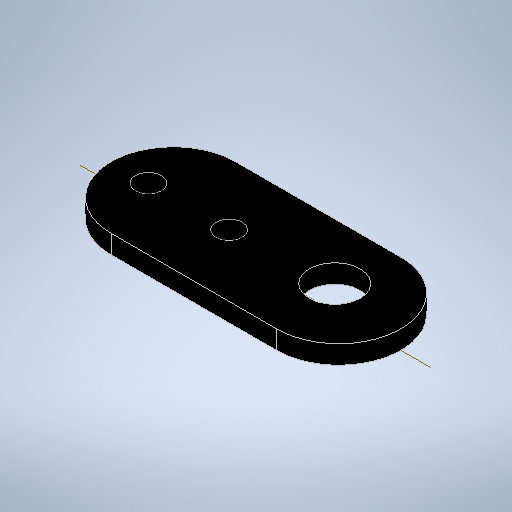
# Autodesk Inventor part: X Adjustment Block
Saved by Autodesk Inventor 2025 (Build 290162000, 162)
## iProperties
Manager: J. Wilburn
Created: 2025-03-12
Part Number: X Adjustment Block
Material: Aluminum 6061
Document SubType Name: Modeling
Designer: MAL16204
Density: 2.7 g/cm^3
Appearance: Anodized - Black
Mass: 6.20979 g
Surface Area: 20.3813 cm^2
Volume: 2.29992 cm^3
Author: Richard Malstrom
Title: X Adjustment Block
Subject: Ender 3 Pro Assembly
Autodesk Inventor part; units mm, degrees
ref_plane "YZ Plane" through (0, 0, 0) normal (1, 0, 0) x (0, 1, 0)
ref_plane "XZ Plane" through (0, 0, 0) normal (0, 1, 0) x (-1, 0, 0)
ref_plane "XY Plane" through (0, 0, 0) normal (0, 0, 1) x (1, 0, 0)
sketch "Sketch1" plane through (0, 0, 0) normal (0, 1, 0) x (-1, 0, 0)
  line L0 (13.325, 0) -> (-13.325, 0) construction
  line L1 (13.325, 10) -> (-13.325, 10)
  line L2 (-13.325, -10) -> (13.325, -10)
  arc A0 (13.325, -10) -> (13.325, 10) centre (13.325, 0) ccw
  arc A1 (-13.325, 10) -> (-13.325, -10) centre (-13.325, 0) ccw
  point P0 (0, 0)
  dimension "d0" = 26.65
  dimension "d1" = 20
  constraints: 8 end point, 4 point on circle, 4 tangent, 2 centre point, 1 horizontal, 1 midpoint, 1 parallel
  measures "d0" distance of L0.end L0.start
  measures "d1" distance between parallel lines of L1 L2
extrude "Extrusion1" add sketch "Sketch1" along normal blind 3
sketch "Sketch2" plane through (0, 3, 0) normal (0, 1, 0) x (1, 0, 0)
  point P0 (0, 0)
  point P1 (-17.33, 0)
  point P2 (-4.33, 0)
  dimension "d4" = 17.33
  dimension "d5" = 4.33
  measures "d4" distance of point (0, 0) point (-17.33, 0)
  measures "d5" distance of point (0, 0) point (-4.33, 0)
hole "Hole1" at (-17.33, 3, 0) at (-4.33, 3, 0) direction (0, -1, 0) diameter 4.2 end through all
sketch "Sketch3" plane through (0, 3, 0) normal (0, 1, 0) x (1, 0, 0)
  line L0 (-32.655, 0) -> (32.655, 0) projected
  point P0 (0, 0)
  point P1 (11.68, 1)
  dimension "d13" = 1
  dimension "d14" = 11.68
  measures "d13" distance from line of L0 point (11.68, 1)
  measures "d14" horizontal distance of point (0, 0) point (11.68, 1)
hole "Hole2" at (11.68, 3, -1) direction (0, -1, 0) diameter 8.2 end through all
body "Solid1"
